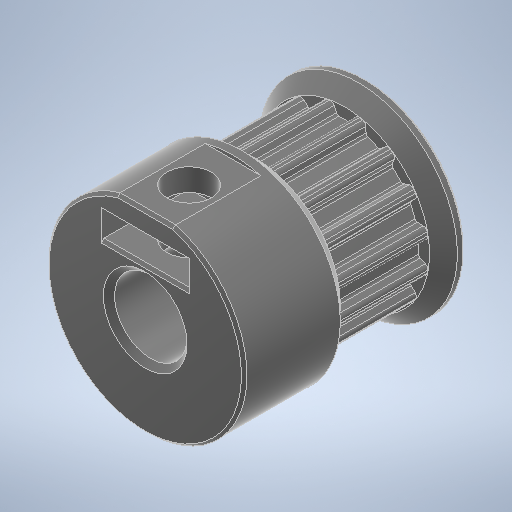
# Autodesk Inventor part: 歯付きプーリ1
Saved by Autodesk Inventor 2025 (Build 290162000, 162)
## iProperties
CustomPartVersion: 1
Created: 2024-06-24
Part Number: 歯付きプーリ1
Material: Steel
Document SubType Name: Modeling
Designer: 8326d
Density: 1 g/cm^3
Appearance: 滑らか - 黒
Author: 8326d
## iProperties of the stored document pully_T2.5-16_3D プリント.ipt
Created: 2024-07-25
Part Number: pully_T2.5-16_3D プリント
Material: 一般
Document SubType Name: Modeling
Designer: 8326d
Density: 1 g/cm^3
Appearance: 既定
Author: 8326d
Autodesk Inventor part; units mm, degrees
ref_plane "YZ Plane" through (0, 0, 0) normal (1, 0, 0) x (0, 1, 0)
ref_plane "XZ Plane" through (0, 0, 0) normal (0, 1, 0) x (-1, 0, 0)
ref_plane "XY Plane" through (0, 0, 0) normal (0, 0, 1) x (1, 0, 0)
sketch "プーリ スケッチ" plane through (0, 0, 0) normal (0, 0, 1) x (1, 0, 0)
  circle A0 centre (0, 0) radius 6.3662 construction
  circle A1 centre (0, 0) radius 6.0662
  circle A2 centre (0, 0) radius 5.3162
  line L0 (-0.847, 6.0068) -> (-0.525, 5.3162)
  line L1 (-0.525, 5.3162) -> (0.525, 5.3162)
  line L2 (0.525, 5.3162) -> (0.847, 6.0068)
  line L3 (0, 0) -> (0, 6.0662) construction
  point P0 (0, 5.3162)
  dimension "d0" = 12.7324
  dimension "d1" = 0.3
  dimension "d2" = 0.75
  dimension "d3" = 50
  dimension "d4" = 1.05
  constraints: 8 end point, 3 coincident, 3 point on circle, 2 centre point, 1 horizontal, 1 midpoint, 1 point on line, 1 vertical, 1 vertical alignment, 3 other
  measures "d0" diameter of A0
  measures "d1" radial gap between concentric circles of A0 A1
  measures "d3" angle of L2 L0
  measures "d4" distance of L0.end L1.end
extrude "基本ボディ" add sketch "プーリ スケッチ" along normal mid plane 6.4 contours A2 | A1 L0 L1 L2 | L2 L1 L0 A1
extrude "歯" cut sketch "プーリ スケッチ" along normal through all both and the other way through all contours L2 L1 L0 A1 picked at (0, 5.8118)
fillet "Fillet" radius 0.2 2 edges at (0.525, 5.3162, 0) (-0.525, 5.3162, 0)
fillet "Fillet" radius 0.3 4 edges at (-0.847, 6.0068, 1.6) (-0.847, 6.0068, -1.6) (0.847, 6.0068, 1.6) (0.847, 6.0068, -1.6)
pattern_circular "Teeth" count 16 over 360 about axis through (0, 0, -10) along (0, 0, 1) of "歯", "Fillet"
sketch "スケッチ2" plane through (0, 0, 3.2) normal (0, 0, 1) x (1, 0, 0)
  circle A0 centre (0, 0) radius 7.1
  dimension "d17" = 14.2
  constraints: 1 centre point, 1 coincident
  measures "d17" diameter of A0
extrude "押し出し3" add sketch "スケッチ2" along normal blind 1.6
chamfer "面取り1" distance 1 angle 45 1 edges at (-7.1, 0, 3.2)
mirror "ミラー1" about plane through (0, 0, 0) normal (0, 0, 1) of "押し出し3", "面取り1"
sketch "スケッチ3" plane through (0, 0, 4.8) normal (0, 0, 1) x (1, 0, 0)
  point P0 (0, 0)
  point P1 (0, 0)
  constraints: 1 coincident
hole "穴1" at (0, 0, 4.8) direction (0, 0, -1) diameter 5.2 end through all
chamfer "面取り2" distance 0.4 angle 45 1 edges at (0, 2.6, -4.8)
chamfer "面取り3" distance 0.2 angle 45 1 edges at (-7.1, 0, -4.8)
sketch "スケッチ4" plane through (0, 0, 4.8) normal (0, 0, 1) x (1, 0, 0)
  circle A0 centre (0, 0) radius 2.6 projected
  circle A1 centre (0, 0) radius 7.1
  line L0 (-2, 6.8125) -> (2, 6.8125)
  circle A2 centre (0, 0) radius 7.1 projected
  dimension "d39" = 4
  constraints: 2 end point, 2 point on circle, 1 centre point, 1 coincident, 1 concentric, 1 horizontal
  measures "d39" distance of L0.start L0.end
extrude "押し出し4" add sketch "スケッチ4" along normal blind 6.3 contours A1 L0 picked at (-0.1045, 5.402)
sketch "スケッチ5" plane through (-2, 6.8125, 4.8) normal (0, 1, 0) x (1, 0, 0)
  line L0 (0, 0) -> (4, 0) projected
  line L1 (0, 0) -> (0, -6.3) projected
  line L2 (4, -6.3) -> (0, -6.3) projected
  line L3 (4, 0) -> (4, -6.3) projected
  line L4 (2, -6.3) -> (2, 0) construction
  line L5 (4, -3.15) -> (0, -3.15) construction
  point P0 (2, 4.8)
  point P1 (2, -3.15)
  constraints: 5 midpoint, 4 end point
hole "穴2" at (0, 6.8125, 7.95) direction (0, -1, 0) diameter 3.2 depth 6
sketch "スケッチ6" plane through (0, 0, 11.1) normal (0, 0, 1) x (1, 0, 0)
  line L0 (-3.15, 3.4125) -> (3.15, 3.4125)
  line L1 (3.15, 3.4125) -> (3.15, 5.2125)
  line L2 (3.15, 5.2125) -> (-3.15, 5.2125)
  line L3 (-3.15, 5.2125) -> (-3.15, 3.4125)
  line L4 (-3.15, 3.4125) -> (3.15, 5.2125) construction
  line L5 (3.15, 3.4125) -> (-3.15, 5.2125) construction
  line L6 (2, 6.8125) -> (-2, 6.8125) projected
  point P0 (0, 0)
  point P1 (0, 4.3125)
  dimension "d47" = 6.3
  dimension "d48" = 1.8
  dimension "d49" = 1.6
  constraints: 12 end point, 2 midpoint, 2 parallel, 1 horizontal, 1 perpendicular, 1 vertical alignment
  measures "d47" distance of L2.end L1.end
  measures "d48" distance of L1.end L0.end
  measures "d49" distance between parallel lines of L6 L2
extrude "押し出し5" cut sketch "スケッチ6" against normal blind 6.3
chamfer "面取り4" distance 0.2 angle 45 2 edges at (0, 5.2125, 11.1) (0, 3.4125, 11.1)
chamfer "面取り5" distance 0.4 angle 45 1 edges at (-2.6, 0, 11.1)
chamfer "面取り6" distance 0.2 angle 45 2 edges at (0, -7.1, 11.1) (0, 6.8125, 11.1)
equation "\"d1\" = da_a"
equation "\"d2\" = da_hg"
equation "\"d3\" = 2 * da_fi"
equation "\"d4\" = da_bw"
equation "\"d5\" = da_bf"
equation "\"d7\" = da_bf"
equation "\"d9\" = da_rb"
equation "\"d10\" = da_rt"
equation "\"da_pb\" = 2.5"
equation "\"da_fi\" = 25deg"
equation "\"da_hg\" = 0.75"
equation "\"da_bw\" = 1.05"
equation "\"da_rb\" = 0.2"
equation "\"da_rt\" = 0.3"
equation "\"da_a\" = 0.3"
equation "\"da_bf\" = 6.4"
equation "\"da_wf\" = 1.5"
equation "\"da_hf\" = 1.5"
body "Solid1"
